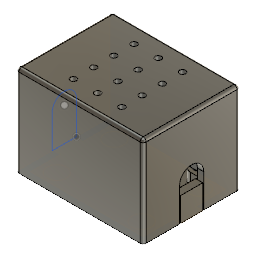
enclosure (Autodesk Fusion 360 design; units mm, degrees)
Autodesk Fusion 360 part; units mm, degrees
sketch "Sketch1" plane through (0, 0, 0) normal (0, 0, 1) x (1, 0, 0) in component "base"
  line L0 (18.6, 13.6) -> (-18.6, 13.6)
  line L1 (-18.6, 13.6) -> (-18.6, -13.6)
  line L2 (-18.6, -13.6) -> (18.6, -13.6)
  line L3 (18.6, -13.6) -> (18.6, 13.6)
  line L4 (18.6, 13.6) -> (-18.6, -13.6) construction
  line L5 (-18.6, 13.6) -> (18.6, -13.6) construction
  circle A0 centre (-14, -9.5) radius 1.6
  circle A1 centre (14, -9.5) radius 1.6
  circle A2 centre (-14, 9.5) radius 1.6
  circle A3 centre (14, 9.5) radius 1.6
  line L6 (0, 13.6) -> (0, -13.6) construction
  line L7 (-18.6, 0) -> (18.6, 0) construction
  dimension "d1" = 37.2
  dimension "d2" = 27.2
  dimension "d3" = 3.2
  dimension "d6" = 28
  dimension "d7" = 19
  dimension "d8" = 9.5
  dimension "d9" = 14
  constraint perpendicular L0 L1
  constraint parallel L0 L2
  constraint parallel L1 L3
  constraint horizontal L0
  constraint coincident L4 origin
  constraint coincident L5 origin
  constraint midpoint L0 L6.start
  constraint midpoint L2 L6.end
  constraint midpoint L1 L7.start
  constraint midpoint L3 L7.end
  measures "d1" distance of L1.end L2.end
  measures "d2" distance of L0.end L1.end
  measures "d3" diameter of A0
  measures "d8" distance of A0.centre L7
  measures "d9" distance of A0.centre L6
extrude "Extrude1" add sketch "Sketch1" along normal blind 2 makes body 1 in component "base"
sketch "Sketch2" plane through (0, 0, 2) normal (0, 0, 1) x (-1, 0, 0) in component "base"
  circle A0 centre (-14, -9.5) radius 1.6
  circle A1 centre (14, -9.5) radius 1.6
  circle A2 centre (14, 9.5) radius 1.6
  circle A3 centre (-14, 9.5) radius 1.6
  line L0 (-18.6, 13.6) -> (-18.6, -13.6)
  line L1 (-18.6, -13.6) -> (18.6, -13.6)
  line L2 (18.6, -13.6) -> (18.6, 13.6)
  line L3 (18.6, 13.6) -> (-18.6, 13.6)
  circle A4 centre (14, -9.5) radius 2.85
  circle A5 centre (-14, -9.5) radius 2.85
  circle A6 centre (-14, 9.5) radius 2.85
  circle A7 centre (14, 9.5) radius 2.85
  line L4 (11.15, -9.5) -> (11.15, -13.6)
  line L5 (14, -6.65) -> (18.6, -6.65)
  line L6 (11.15, 9.5) -> (11.15, 13.6)
  line L7 (14, 6.65) -> (18.6, 6.65)
  line L8 (-14, 6.65) -> (-18.6, 6.65)
  line L9 (-11.15, 9.5) -> (-11.15, 13.6)
  line L10 (-14, -6.65) -> (-18.6, -6.65)
  line L11 (-11.15, -9.5) -> (-11.15, -13.6)
  dimension "d12" = 5.7
  dimension "d13" = 5.7
  dimension "d14" = 5.7
  dimension "d15" = 5.7
  constraint concentric A1 A4
  constraint concentric A0 A5
  constraint concentric A3 A6
  constraint concentric A2 A7
  constraint coincident A4 L4.start
  constraint coincident L1 L4.end
  constraint perpendicular L1 L4
  constraint coincident A4 L5.start
  constraint coincident L2 L5.end
  constraint perpendicular L2 L5
  constraint coincident A7 L6.start
  constraint coincident L3 L6.end
  constraint perpendicular L3 L6
  constraint coincident A7 L7.start
  constraint tangent A7 L7
  constraint perpendicular L6 L7
  constraint coincident A6 L8.start
  constraint coincident L0 L8.end
  constraint perpendicular L0 L8
  constraint coincident A6 L9.start
  constraint coincident L3 L9.end
  constraint perpendicular L3 L9
  constraint coincident A5 L10.start
  constraint coincident L0 L10.end
  constraint perpendicular L0 L10
  constraint coincident A5 L11.start
  constraint coincident L1 L11.end
  constraint perpendicular L1 L11
  constraint tangent A6 L8
  constraint tangent A6 L9
  constraint tangent A5 L10
  constraint tangent A5 L11
  constraint tangent A4 L4
  constraint tangent A4 L5
  constraint tangent A7 L6
  measures "d12" diameter of A4
  measures "d13" diameter of A5
  measures "d14" diameter of A6
  measures "d15" diameter of A7
extrude "Extrude2" add sketch "Sketch2" along normal blind 4 contours L0 L3 A6 L8 L9 | L0 L1 A5 L10 L11 | A6 | L2 L3 A7 L6 L7 | A5 | A7 | L1 L2 A4 L4 L5 | A4 bodies 1 in component "base"
sketch "Sketch1 (2)" plane through (0, 0, 0) normal (0, 0, 1) x (1, 0, 0) in component "cover"
  line L0 (21, 16) -> (-21, 16)
  line L1 (-21, 16) -> (-21, -16)
  line L2 (-21, -16) -> (21, -16)
  line L3 (21, -16) -> (21, 16)
  line L4 (21, 16) -> (-21, -16) construction
  line L5 (-21, 16) -> (21, -16) construction
  dimension "d18" = 32
  dimension "d19" = 42
  constraint perpendicular L0 L1
  constraint parallel L0 L2
  constraint parallel L1 L3
  constraint horizontal L0
  constraint coincident L4 origin
  constraint coincident L5 origin
  measures "d18" distance of L0.end L1.end
  measures "d19" distance of L1 L3
extrude "Extrude1'" add sketch "Sketch1 (2)" along normal blind 30 separate body makes body 2 in component "cover"
shell "Shell1" thickness 2.08 removed faces 1 at (-7, 5.3333, 0) on bodies 2 in component "cover"
sketch "Sketch2 (2)" plane through (0, 0, 30) normal (0, 0, 1) x (-1, 0, 0) in component "cover"
  line L0 (-21, 16) -> (-21, -16)
  line L1 (-21, -16) -> (21, -16)
  line L2 (21, -16) -> (21, 16)
  line L3 (21, 16) -> (-21, 16)
  circle A0 centre (14, 9.5) radius 2.85
  circle A1 centre (-14, 9.5) radius 2.85
  circle A2 centre (-14, -9.5) radius 2.85
  circle A3 centre (14, -9.5) radius 2.85
  circle A4 centre (-14, -9.5) radius 1.3
  circle A5 centre (-14, 9.5) radius 1.3
  circle A6 centre (14, 9.5) radius 1.3
  circle A7 centre (14, -9.5) radius 1.3
  line L4 (-11.15, 9.5) -> (-11.15, 16)
  line L5 (-14, 6.65) -> (-21, 6.65)
  line L6 (-18.92, 13.92) -> (-18.92, -13.92)
  line L7 (-11.15, -9.5) -> (-11.15, -16)
  line L8 (11.15, -9.5) -> (11.15, -16)
  line L9 (14, -6.65) -> (21, -6.65)
  line L10 (11.15, 9.5) -> (11.15, 16)
  line L11 (18.92, -13.92) -> (18.92, 13.92)
  line L12 (14, 6.65) -> (21, 6.65)
  line L13 (-14, -6.65) -> (-21, -6.65)
  dimension "d23" = 2.6
  dimension "d24" = 2.6
  dimension "d25" = 2.6
  dimension "d26" = 2.6
  constraint concentric A2 A4
  constraint concentric A1 A5
  constraint concentric A0 A6
  constraint concentric A3 A7
  constraint coincident A1 L4.start
  constraint coincident L3 L4.end
  constraint perpendicular L3 L4
  constraint coincident A1 L5.start
  constraint coincident L0 L5.end
  constraint perpendicular L0 L5
  constraint coincident A2 L7.start
  constraint coincident L1 L7.end
  constraint perpendicular L1 L7
  constraint coincident A3 L8.start
  constraint coincident L1 L8.end
  constraint perpendicular L1 L8
  constraint coincident A3 L9.start
  constraint coincident L2 L9.end
  constraint perpendicular L2 L9
  constraint coincident A0 L10.start
  constraint coincident L3 L10.end
  constraint perpendicular L3 L10
  constraint coincident A0 L12.start
  constraint perpendicular L11 L12
  constraint tangent A1 L4
  constraint tangent A1 L5
  constraint tangent A2 L7
  constraint tangent A3 L8
  constraint tangent A3 L9
  constraint tangent A0 L10
  constraint tangent A0 L12
  constraint coincident A2 L13.start
  constraint coincident L0 L13.end
  constraint perpendicular L0 L13
  constraint tangent A2 L13
  measures "d23" diameter of A4
  measures "d24" diameter of A5
  measures "d25" diameter of A6
  measures "d26" diameter of A7
extrude "Extrude2'" add sketch "Sketch2 (2)" against normal blind 22.5 contours L0 L3 A1 L4 L5 | L0 L1 A2 L7 L13 | L2 L3 A0 L10 L12 | A1 | A0 | A2 | L1 L2 A3 L8 L9 | A3 bodies 2 in component "cover"
fillet "Fillet2" radius 1 8 edges at (-21, -16, 15) (21, -16, 15) (0, -16, 30) (21, 0, 30) (-21, 0, 30) (21, 16, 15) (0, 16, 30) (-21, 16, 15) on bodies 2 in component "cover"
chamfer "Chamfer1" distance 1.6 angle 45 4 edges at (-15.4917, -8.9214, 0) (12.5083, -8.9214, 0) (12.5083, 10.0786, 0) (-15.4917, 10.0786, 0) on bodies 1 in component "base"
sketch "Sketch3" plane through (-21, 0, 0) normal (-1, 0, 0) x (0, -1, 0) in component "cover"
  line L0 (-15, 29) -> (-15, 0)
  line L1 (-15, 0) -> (15, 0)
  line L2 (15, 0) -> (15, 29)
  line L3 (15, 29) -> (-15, 29)
  line L4 (4, 8) -> (4, 11)
  line L5 (-4, 11) -> (-4, 8)
  arc A0 (4, 11) -> (-4, 11) centre (0, 11) ccw
  line L6 (-4, 8) -> (-4, 0)
  line L7 (4, 8) -> (4, 0)
  line L8 (4, 0) -> (-4, 0)
  dimension "d33" = 8
  dimension "d35" = 3
  constraint vertical L4
  constraint vertical L5
  constraint coincident L1 L6.end
  constraint perpendicular L7 L8
  measures "d33" distance of L1 L4.start
  measures "d35" distance of L4.start L4.end
extrude "Extrude3" cut sketch "Sketch3" against normal through all contours L1 L4 L5 A0 L6 L7 L8 bodies 2 in component "cover"
sketch "Sketch3 (2)" plane through (0, 0, 0) normal (0, 0, -1) x (1, 0, 0) in component "base"
  circle A0 centre (14, -9.5) radius 3.2
  circle A1 centre (-14, 9.5) radius 3.2
  line L0 (18.6, -13.6) -> (18.6, 13.6)
  line L1 (18.6, 13.6) -> (-18.6, 13.6)
  line L2 (-18.6, 13.6) -> (-18.6, -13.6)
  line L3 (-18.6, -13.6) -> (18.6, -13.6)
  circle A2 centre (14, 9.5) radius 3.2
  circle A3 centre (-14, -9.5) radius 3.2
  line L4 (21, -3.68) -> (-21, -3.68)
  line L5 (-21, -3.68) -> (-21, 3.68)
  line L6 (-21, 3.68) -> (21, 3.68)
  line L7 (21, 3.68) -> (21, -3.68)
  line L8 (21, -3.68) -> (-21, 3.68) construction
  line L9 (-21, -3.68) -> (21, 3.68) construction
  line L10 (21, 4) -> (21, -4)
  line L11 (21, -4) -> (18.92, -4)
  dimension "d36" = 0.32
  constraint perpendicular L4 L5
  constraint parallel L4 L6
  constraint parallel L5 L7
  constraint horizontal L4
  constraint coincident L4.start L10
  constraint coincident L8 origin
  constraint coincident L9 origin
  measures "d36" distance of L4 L11
extrude "Extrude3'" add sketch "Sketch3 (2)" against normal blind 8 contours L0 L4 L6 L7 L10 | L2 L4 L5 L6 bodies 1 in component "base"
sketch "Sketch4" plane through (0, 0, 30) normal (0, 0, 1) x (-1, 0, 0) in component "cover"
  line L0 (-20, 15) -> (-20, -15)
  line L1 (-20, -15) -> (20, -15)
  line L2 (20, -15) -> (20, 15)
  line L3 (20, 15) -> (-20, 15)
  circle A0 centre (8, -10) radius 1
  circle A1 centre (0, -10) radius 1
  circle A2 centre (-8, -10) radius 1
  circle A3 centre (8, -3.3333) radius 1
  circle A4 centre (0, -3.3333) radius 1
  circle A5 centre (-8, -3.3333) radius 1
  circle A6 centre (8, 3.3333) radius 1
  circle A7 centre (0, 3.3333) radius 1
  circle A8 centre (-8, 3.3333) radius 1
  circle A9 centre (8, 10) radius 1
  circle A10 centre (0, 10) radius 1
  circle A11 centre (-8, 10) radius 1
  dimension "d40" = 2
  dimension "d43" = -16
  dimension "d44" = 20
  measures "d40" diameter of A0
extrude "Extrude4" cut sketch "Sketch4" against normal up to surface (2.08 mm away) contours A0 | A1 | A2 | A3 | A4 | A5 | A6 | A7 | A8 | A9 | A10 | A11 bodies 2 in component "cover"
sketch "Sketch5" plane through (0, 0, 2) normal (0, 0, 1) x (-1, 0, 0) in component "base"
  line L0 (18.6, 6.65) -> (14, 6.65)
  arc A0 (11.15, 9.5) -> (14, 6.65) centre (14, 9.5) ccw
  line L1 (11.15, 9.5) -> (11.15, 13.6)
  line L2 (11.15, 13.6) -> (-11.15, 13.6)
  line L3 (-11.15, 13.6) -> (-11.15, 9.5)
  arc A1 (-14, 6.65) -> (-11.15, 9.5) centre (-14, 9.5) ccw
  line L4 (-14, 6.65) -> (-18.6, 6.65)
  line L5 (-18.6, 6.65) -> (-18.6, 3.68)
  line L6 (-18.6, 3.68) -> (-18.6, -3.68)
  line L7 (-18.6, -3.68) -> (-18.6, -6.65)
  line L8 (-18.6, -6.65) -> (-14, -6.65)
  arc A2 (-11.15, -9.5) -> (-14, -6.65) centre (-14, -9.5) ccw
  line L9 (-11.15, -9.5) -> (-11.15, -13.6)
  line L10 (-11.15, -13.6) -> (11.15, -13.6)
  line L11 (11.15, -13.6) -> (11.15, -9.5)
  arc A3 (14, -6.65) -> (11.15, -9.5) centre (14, -9.5) ccw
  line L12 (14, -6.65) -> (18.6, -6.65)
  line L13 (18.6, -6.65) -> (18.6, -3.68)
  line L14 (18.6, -3.68) -> (18.6, 3.68)
  line L15 (18.6, 3.68) -> (18.6, 6.65)
  line L16 (17.74, -12.74) -> (-17.74, -12.74)
  line L17 (-17.74, -12.74) -> (-17.74, 12.74)
  line L18 (-17.74, 12.74) -> (17.74, 12.74)
  line L19 (17.74, 12.74) -> (17.74, -12.74)
  line L20 (18.6, 13.6) -> (-18.6, 13.6)
  line L21 (-18.6, 13.6) -> (-18.6, 3.68)
  line L22 (-18.6, -3.68) -> (-18.6, -13.6)
  line L23 (-18.6, -13.6) -> (18.6, -13.6)
  line L24 (18.6, -13.6) -> (18.6, -3.68)
  line L25 (18.6, 3.68) -> (18.6, 13.6)
  dimension "d53" = 0.86
  dimension "d54" = 0.86
  dimension "d55" = 0.86
  dimension "d56" = 0.86
  constraint horizontal L16
  constraint vertical L17
  constraint horizontal L18
  constraint vertical L19
  measures "d53" distance of L10 L16
  measures "d54" distance of L2 L18
  measures "d55" distance of L14 L19
  measures "d56" distance of L7 L17
extrude "Extrude5" add sketch "Sketch5" along normal blind 5 contours L0 L12 L13 L14 L15 L19 L24 L25 | L0 L1 L18 L19 L20 L25 | L11 L12 L16 L19 L23 L24 | L1 L2 L3 L18 L20 | L3 L4 L17 L18 L20 L21 | L9 L10 L11 L16 L23 | L8 L9 L16 L17 L22 L23 | L4 L5 L6 L7 L8 L17 L21 L22 bodies 1 in component "base"
fillet "Fillet4" radius 1 2 edges at (-18.6, 0, 7) (18.6, 0, 7) on bodies 1 in component "base"
sketch "Sketch6" plane through (0, 0, 0) normal (0, 0, -1) x (1, 0, 0) in component "base"
  circle A0 centre (14, -9.5) radius 3.2
  circle A1 centre (-14, 9.5) radius 3.2
  line L0 (18.6, 3.68) -> (18.6, 13.6)
  line L1 (18.6, 13.6) -> (-18.6, 13.6)
  line L2 (-18.6, 13.6) -> (-18.6, 3.68)
  line L3 (-18.6, 3.68) -> (-21, 3.68)
  line L4 (-21, 3.68) -> (-21, -3.68)
  line L5 (-21, -3.68) -> (-18.6, -3.68)
  line L6 (-18.6, -3.68) -> (-18.6, -13.6)
  line L7 (-18.6, -13.6) -> (18.6, -13.6)
  line L8 (18.6, -13.6) -> (18.6, -3.68)
  line L9 (18.6, -3.68) -> (21, -3.68)
  line L10 (21, -3.68) -> (21, 3.68)
  line L11 (21, 3.68) -> (18.6, 3.68)
  circle A2 centre (14, 9.5) radius 3.2
  circle A3 centre (-14, -9.5) radius 3.2
component "base" placed x (1, 0, 0) y (0, 1, 0) z (0, 0, 1) at (0, 0, 0)
component "cover" placed x (1, 0, 0) y (0, 1, 0) z (0, 0, 1) at (0, 0, 0)
equation "d8 = ( 19 / 2 ) * 1 mm"
equation "d9 = ( 28 / 2 ) * 1 mm"
equation "d13 = d12"
equation "d14 = d12"
equation "d15 = d12"
equation "d24 = d23"
equation "d25 = d23"
equation "d26 = d23"
equation "d54 = d53"
equation "d55 = d53"
equation "d56 = d53"
